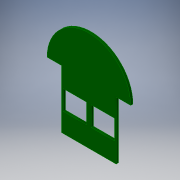
# Autodesk Inventor part: Micromouse_pcb
Saved by Autodesk Inventor 2018 (Build 220112000, 112)
## iProperties
Created: 2017-09-20
Part Number: Micromouse_pcb
Material: Generic
Document SubType Name: Modeling
Designer: test
Density: 1 g/cm^3
Appearance: Board Outline
Author: test
Autodesk Inventor part; units mm, degrees
ref_plane "YZ Plane" through (0, 0, 0) normal (1, 0, 0) x (0, 1, 0)
ref_plane "XZ Plane" through (0, 0, 0) normal (0, 1, 0) x (-1, 0, 0)
ref_plane "XY Plane" through (0, 0, 0) normal (0, 0, 1) x (1, 0, 0)
sketch "Sketch1" plane through (0, 0, 0) normal (0, 0, 1) x (1, 0, 0)
  line L0 (-36, 50) -> (-23.5, 50)
  line L1 (-23.5, 50) -> (-23.5, 0)
  line L2 (-23.5, 0) -> (0, 0)
  arc A0 (0, 86) -> (-36, 50) centre (0, 50) ccw
  line L3 (0, 0) -> (0, 227.422)
  line L4 (0, 50) -> (-63.2946, 50) construction
  line L5 (36, 50) -> (23.5, 50)
  line L6 (23.5, 50) -> (23.5, 0)
  line L7 (23.5, 0) -> (0, 0)
  arc A1 (36, 50) -> (0, 86) centre (0, 50) ccw
  point P0 (0, 0)
  dimension "d4" = 36
  dimension "d5" = 50
  dimension "d6" = 47
  constraints: 16 end point, 4 point on circle, 3 point on line, 3 symmetric about line, 2 centre point, 2 horizontal, 2 vertical, 1 coincident, 1 collinear, 1 other
  measures "d4" radius of A0
  measures "d5" distance from line of L2 L4.start
  measures "d6" diameter of L1 L3
extrude "Micromouse1.2.kicad_pcb_Outline" add sketch "Sketch1" along normal blind 2
sketch "Sketch3" plane through (0, 0, 2) normal (0, 0, 1) x (1, 0, 0)
  line L0 (-23.5, 0) -> (23.5, 0) projected
  line L1 (23.5, 0) -> (23.5, 50) projected
  line L2 (23.5, 50) -> (36, 50) projected
  arc A0 (36, 50) -> (-36, 50) centre (0, 50) ccw projected
  line L3 (-36, 50) -> (-23.5, 50) projected
  line L4 (-23.5, 50) -> (-23.5, 0) projected
  line L5 (-57.2581, 25) -> (65.9372, 25)
  line L6 (0, 50) -> (0, -46.1681)
  line L7 (-22, 33.5) -> (-2, 33.5)
  line L8 (-2, 33.5) -> (-2, 16.5)
  line L9 (-2, 16.5) -> (-22, 16.5)
  line L10 (-22, 16.5) -> (-22, 33.5)
  line L11 (22, 33.5) -> (2, 33.5)
  line L12 (2, 33.5) -> (2, 16.5)
  line L13 (2, 16.5) -> (22, 16.5)
  line L14 (22, 16.5) -> (22, 33.5)
  point P0 (0, 0)
  point P1 (-30, 25)
  point P2 (-2, 25)
  dimension "d7" = 25
  dimension "d8" = 17
  dimension "d9" = 20
  dimension "d10" = 4
  constraints: 20 end point, 4 symmetric about line, 2 horizontal, 2 parallel, 2 point on line, 1 midpoint, 1 perpendicular, 1 vertical
  measures "d7" distance between parallel lines of L5 L3
  measures "d8" distance between parallel lines of L9 L7
  measures "d9" distance between parallel lines of L8 L10
  measures "d10" diameter of L8 L6
extrude "Extrusion3" cut sketch "Sketch3" against normal through all contours L10 L7 L8 L5 | L5 L8 L9 L10 | L12 L11 L14 L5 | L5 L14 L13 L12
sketch "Sketch4" plane through (0, 0, 2) normal (0, 0, 1) x (1, 0, 0)
  line L0 (-22, 16.5) -> (-22, 33.5) projected
  line L1 (-22, 33.5) -> (-2, 33.5) projected
  line L2 (-2, 33.5) -> (-2, 16.5) projected
  line L3 (-2, 16.5) -> (-22, 16.5) projected
  line L4 (22, 33.5) -> (22, 16.5) projected
  line L5 (22, 16.5) -> (2, 16.5) projected
  line L6 (2, 16.5) -> (2, 33.5) projected
  line L7 (2, 33.5) -> (22, 33.5) projected
  line L8 (-23.5, 0) -> (23.5, 0) projected
  line L9 (23.5, 0) -> (23.5, 50) projected
  line L10 (23.5, 50) -> (36, 50) projected
  arc A0 (36, 50) -> (-36, 50) centre (0, 50) ccw projected
  line L11 (-36, 50) -> (-23.5, 50) projected
  line L12 (-23.5, 50) -> (-23.5, 0) projected
  circle A1 centre (-26, 40) radius 0.5
  line L13 (0, 50) -> (0, -21.7733)
  line L14 (-26, 40) -> (-26, -11.7525) construction
  line L15 (-22, 16.5) -> (-22, 33.5) projected
  line L16 (-22, 25) -> (-54.7599, 25)
  circle A2 centre (-26, 10) radius 0.5
  circle A3 centre (26, 40) radius 0.5
  circle A4 centre (26, 10) radius 0.5
  point P0 (0, 0)
  dimension "d13" = 1
  dimension "d14" = 52
  dimension "d17" = 30
  constraints: 6 end point, 4 centre point, 3 symmetric about line, 2 vertical, 1 coincident, 1 horizontal, 1 midpoint, 3 other
  measures "d13" diameter of A1
  measures "d14" diameter of L14.start L13
  measures "d17" diameter of L14.start L16
extrude "Extrusion4" cut sketch "Sketch4" against normal through all contours A1 | A2 | A3 | A4
hole "Hole1" [suppressed]
hole "Hole2" [suppressed]
hole "Hole3" [suppressed]
hole "Hole4" [suppressed]
body "Solid1"
